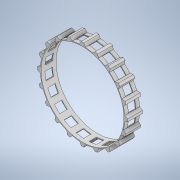
# Autodesk Inventor part: tracks_v1
Saved by Autodesk Inventor 2020 (Build 240168000, 168)
## iProperties
Created: 2020-04-20
Part Number: tracks_v1
Material: Ogólny
Document SubType Name: Modeling
Designer: blep
Density: 1 g/cm^3
Appearance: Domyślna
Author: blep
Autodesk Inventor part; units mm, degrees
ref_plane "XZ Plane" through (0, 0, 0) normal (0, 1, 0) x (-1, 0, 0)
ref_plane "XY Plane" through (0, 0, 0) normal (0, 0, 1) x (1, 0, 0)
sketch "Szkic1" plane through (0, 0, 0) normal (0, 0, 1) x (1, 0, 0)
  circle A0 centre (0, 0) radius 55.5545
  circle A1 centre (0, 0) radius 56.5545
  dimension "d0" = 111.109
  dimension "d1" = 1
  constraints: 2 centre point, 1 coincident
  measures "d0" diameter of A0
  measures "d1" radial gap between concentric circles of A0 A1
extrude "Wyciągnięcie proste1" add sketch "Szkic1" along normal blind 20
ref_plane "Płaszczyzna konstrukcyjna1" through (56.5545, 0, 0) normal (1, 0, 0) x (0, 1, 0)
sketch "Szkic2" plane through (56.5545, 0, 0) normal (1, 0, 0) x (0, 1, 0)
  line L0 (56.5545, 0) -> (-56.5545, 0)
  line L1 (56.5545, 20) -> (-56.5545, 20) projected
  line L2 (-3.764, 0) -> (3.764, 0)
  line L3 (3.764, 0) -> (3.764, 20)
  line L4 (3.764, 20) -> (-3.764, 20)
  line L5 (-3.764, 20) -> (-3.764, 0)
  line L6 (56.5545, 0) -> (-56.5545, 0) construction
  line L7 (-3.764, 20) -> (-56.5545, 0) construction
  line L8 (3.764, 20) -> (56.5545, 0) construction
  point P0 (-3.764, 20)
  point P1 (3.764, 0)
  dimension "d4" = 7.528
  constraints: 14 end point, 2 parallel, 1 equal length, 1 horizontal, 1 perpendicular, 1 point on line
  measures "d4" distance between parallel lines of L3 L5
extrude "Wyciągnięcie proste2" add sketch "Szkic2" along normal blind 4 and the other way blind 1
chamfer "Faza1" distance 2 distance2 4 1 edges at (60.5545, 3.764, 10) measured on face at (60.5545, -1.2547, 6.6667)
chamfer "Faza2" distance 2 distance2 4 1 edges at (60.5545, -3.764, 10) measured on face at (60.5545, -1.9213, 13.3333)
pattern_circular "Szyk kołowy1" count 20 over 360 about axis through (0, 0, 0) along (0, 0, 1) of "Wyciągnięcie proste2", "Faza1", "Faza2"
sketch "Szkic3" plane through (0, 0, 20) normal (0, 0, 1) x (1, 0, 0)
  line L0 (56.4291, -3.764) -> (55.4356, -3.6332)
  line L1 (54.8304, -13.8578) -> (53.8609, -13.6127)
  line L2 (0.2459, 3.6325) -> (56.4291, -3.764) construction
  line L3 (54.8304, -13.8578) -> (0, 0) construction
  arc A0 (53.8609, -13.6127) -> (55.4356, -3.6332) centre (0, 0) ccw
  arc A1 (54.8304, -13.8578) -> (56.4291, -3.764) centre (0, 0) ccw
  circle A2 centre (0, 0) radius 55.5545 construction
  line L4 (54.8304, 13.8578) -> (53.8451, 13.6752)
  line L5 (56.4291, 3.764) -> (55.4313, 3.6974)
  arc A3 (55.4313, 3.6974) -> (53.8451, 13.6752) centre (0, 0) ccw
  arc A4 (56.4291, 3.764) -> (54.8304, 13.8578) centre (0, 0) ccw
  line L6 (47.8645, 30.1231) -> (46.9839, 29.6449)
  line L7 (52.5041, 21.0173) -> (51.5757, 20.6457)
  arc A5 (51.5757, 20.6457) -> (46.9839, 29.6449) centre (0, 0) ccw
  arc A6 (52.5041, 21.0173) -> (47.8645, 30.1231) centre (0, 0) ccw
  line L8 (36.2133, 43.4397) -> (35.5235, 42.7128)
  line L9 (43.4397, 36.2133) -> (42.6716, 35.573)
  arc A7 (42.6716, 35.573) -> (35.5235, 42.7128) centre (0, 0) ccw
  arc A8 (43.4397, 36.2133) -> (36.2133, 43.4397) centre (0, 0) ccw
  line L10 (21.0173, 52.5041) -> (20.5859, 51.5996)
  line L11 (30.1231, 47.8645) -> (29.5904, 47.0182)
  arc A9 (29.5904, 47.0182) -> (20.5859, 51.5996) centre (0, 0) ccw
  arc A10 (30.1231, 47.8645) -> (21.0173, 52.5041) centre (0, 0) ccw
  line L12 (3.764, 56.4291) -> (3.6332, 55.4356)
  line L13 (13.8578, 54.8304) -> (13.6127, 53.8609)
  arc A11 (13.6127, 53.8609) -> (3.6332, 55.4356) centre (0, 0) ccw
  arc A12 (13.8578, 54.8304) -> (3.764, 56.4291) centre (0, 0) ccw
  line L14 (-13.8578, 54.8304) -> (-13.6752, 53.8451)
  line L15 (-3.764, 56.4291) -> (-3.6974, 55.4313)
  arc A13 (-3.6974, 55.4313) -> (-13.6752, 53.8451) centre (0, 0) ccw
  arc A14 (-3.764, 56.4291) -> (-13.8578, 54.8304) centre (0, 0) ccw
  line L16 (-30.1231, 47.8645) -> (-29.6449, 46.9839)
  line L17 (-21.0173, 52.5041) -> (-20.6457, 51.5757)
  arc A15 (-20.6457, 51.5757) -> (-29.6449, 46.9839) centre (0, 0) ccw
  arc A16 (-21.0173, 52.5041) -> (-30.1231, 47.8645) centre (0, 0) ccw
  line L18 (-43.4397, 36.2133) -> (-42.7128, 35.5235)
  line L19 (-36.2133, 43.4397) -> (-35.573, 42.6716)
  arc A17 (-35.573, 42.6716) -> (-42.7128, 35.5235) centre (0, 0) ccw
  arc A18 (-36.2133, 43.4397) -> (-43.4397, 36.2133) centre (0, 0) ccw
  line L20 (-52.5041, 21.0173) -> (-51.5996, 20.5859)
  line L21 (-47.8645, 30.1231) -> (-47.0182, 29.5904)
  arc A19 (-47.0182, 29.5904) -> (-51.5996, 20.5859) centre (0, 0) ccw
  arc A20 (-47.8645, 30.1231) -> (-52.5041, 21.0173) centre (0, 0) ccw
  line L22 (-56.4291, 3.764) -> (-55.4356, 3.6332)
  line L23 (-54.8304, 13.8578) -> (-53.8609, 13.6127)
  arc A21 (-53.8609, 13.6127) -> (-55.4356, 3.6332) centre (0, 0) ccw
  arc A22 (-54.8304, 13.8578) -> (-56.4291, 3.764) centre (0, 0) ccw
  line L24 (-54.8304, -13.8578) -> (-53.8451, -13.6752)
  line L25 (-56.4291, -3.764) -> (-55.4313, -3.6974)
  arc A23 (-55.4313, -3.6974) -> (-53.8451, -13.6752) centre (0, 0) ccw
  arc A24 (-56.4291, -3.764) -> (-54.8304, -13.8578) centre (0, 0) ccw
  line L26 (-47.8645, -30.1231) -> (-46.9839, -29.6449)
  line L27 (-52.5041, -21.0173) -> (-51.5757, -20.6457)
  arc A25 (-51.5757, -20.6457) -> (-46.9839, -29.6449) centre (0, 0) ccw
  arc A26 (-52.5041, -21.0173) -> (-47.8645, -30.1231) centre (0, 0) ccw
  line L28 (-36.2133, -43.4397) -> (-35.5235, -42.7128)
  line L29 (-43.4397, -36.2133) -> (-42.6716, -35.573)
  arc A27 (-42.6716, -35.573) -> (-35.5235, -42.7128) centre (0, 0) ccw
  arc A28 (-43.4397, -36.2133) -> (-36.2133, -43.4397) centre (0, 0) ccw
  line L30 (-21.0173, -52.5041) -> (-20.5859, -51.5996)
  line L31 (-30.1231, -47.8645) -> (-29.5904, -47.0182)
  arc A29 (-29.5904, -47.0182) -> (-20.5859, -51.5996) centre (0, 0) ccw
  arc A30 (-30.1231, -47.8645) -> (-21.0173, -52.5041) centre (0, 0) ccw
  line L32 (-3.764, -56.4291) -> (-3.6332, -55.4356)
  line L33 (-13.8578, -54.8304) -> (-13.6127, -53.8609)
  arc A31 (-13.6127, -53.8609) -> (-3.6332, -55.4356) centre (0, 0) ccw
  arc A32 (-13.8578, -54.8304) -> (-3.764, -56.4291) centre (0, 0) ccw
  line L34 (13.8578, -54.8304) -> (13.6752, -53.8451)
  line L35 (3.764, -56.4291) -> (3.6974, -55.4313)
  arc A33 (3.6974, -55.4313) -> (13.6752, -53.8451) centre (0, 0) ccw
  arc A34 (3.764, -56.4291) -> (13.8578, -54.8304) centre (0, 0) ccw
  line L36 (30.1231, -47.8645) -> (29.6449, -46.9839)
  line L37 (21.0173, -52.5041) -> (20.6457, -51.5757)
  arc A35 (20.6457, -51.5757) -> (29.6449, -46.9839) centre (0, 0) ccw
  arc A36 (21.0173, -52.5041) -> (30.1231, -47.8645) centre (0, 0) ccw
  line L38 (43.4397, -36.2133) -> (42.7128, -35.5235)
  line L39 (36.2133, -43.4397) -> (35.573, -42.6716)
  arc A37 (35.573, -42.6716) -> (42.7128, -35.5235) centre (0, 0) ccw
  arc A38 (36.2133, -43.4397) -> (43.4397, -36.2133) centre (0, 0) ccw
  line L40 (52.5041, -21.0173) -> (51.5996, -20.5859)
  line L41 (47.8645, -30.1231) -> (47.0182, -29.5904)
  arc A39 (47.0182, -29.5904) -> (51.5996, -20.5859) centre (0, 0) ccw
  arc A40 (47.8645, -30.1231) -> (52.5041, -21.0173) centre (0, 0) ccw
  point P0 (48.6753, 30.7121)
  point P1 (36.8024, 44.2505)
  point P2 (21.327, 53.4573)
  point P3 (3.764, 57.4313)
  point P4 (-14.1675, 55.7835)
  point P5 (-30.7121, 48.6753)
  point P6 (-44.2505, 36.8024)
  point P7 (-53.4573, 21.327)
  point P8 (-57.4313, 3.764)
  point P9 (-55.7835, -14.1675)
  point P10 (-48.6753, -30.7121)
  point P11 (-36.8024, -44.2505)
  point P12 (-21.327, -53.4573)
  point P13 (-3.764, -57.4313)
  point P14 (14.1675, -55.7835)
  point P15 (30.7121, -48.6753)
  point P16 (44.2505, -36.8024)
  point P17 (53.4573, -21.327)
  point P18 (57.4313, -3.764)
  point P19 (55.7835, 14.1675)
  point P20 (-54.8304, -13.8578)
  point P21 (-36.2133, -43.4397)
  point P22 (-21.0173, -52.5041)
  point P23 (-3.764, -56.4291)
  point P24 (13.8578, -54.8304)
  point P25 (30.1231, -47.8645)
  point P26 (52.5041, -21.0173)
  point P27 (21.0173, 52.5041)
  point P28 (3.764, 56.4291)
  point P29 (-43.4397, 36.2133)
  dimension "d22" = 360
  constraints: 84 end point, 80 point on circle, 41 coincident, 40 centre point, 2 collinear, 1 concentric, 1 point on line, 222 other
extrude "Wyciągnięcie proste3" cut sketch "Szkic3" against normal blind 15
extrude "Wyciągnięcie proste4" add sketch "Szkic3" against normal blind 5
